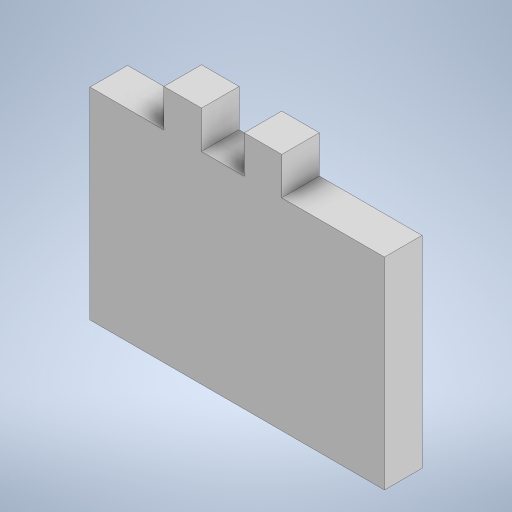
# Autodesk Inventor part: casterholderA
Saved by Autodesk Inventor 2023.2 (Build 272271000, 271)
## iProperties
Created: 2024-08-15
Part Number: casterholderA
Material: Generic
Document SubType Name: Modeling
Designer: PC
Density: 1 g/cm^3
Appearance: Default
Author: PC
Autodesk Inventor part; units mm, degrees
ref_plane "YZ Plane" through (0, 0, 0) normal (1, 0, 0) x (0, 1, 0)
ref_plane "XZ Plane" through (0, 0, 0) normal (0, 1, 0) x (-1, 0, 0)
ref_plane "XY Plane" through (0, 0, 0) normal (0, 0, 1) x (1, 0, 0)
sketch "Sketch1" plane through (0, 0, 0) normal (0, 0, 1) x (1, 0, 0)
  line L0 (20, -16.25) -> (-20, -16.25)
  line L1 (-20, -16.25) -> (-20, 16.25)
  line L2 (-20, 16.25) -> (20, 16.25)
  line L3 (20, 16.25) -> (20, -16.25)
  line L4 (20, -16.25) -> (-20, 16.25) construction
  line L5 (-20, -16.25) -> (20, 16.25) construction
  point P0 (0, 0)
  dimension "d0" = 40
  dimension "d1" = 32.5
  constraints: 12 end point, 2 midpoint, 2 parallel, 1 horizontal, 1 perpendicular
  measures "d0" distance of L1.end L2.end
  measures "d1" distance of L0.end L1.end
extrude "Extrusion1" add sketch "Sketch1" along normal blind 5.1
sketch "Sketch2" plane through (0, 0, 5.1) normal (0, 0, 1) x (1, 0, 0)
  line L0 (-20, 16.25) -> (-20, -16.25) projected
  line L1 (-20, 16.25) -> (-9.95, 16.25)
  line L2 (-9.95, 16.25) -> (-9.95, 11.15)
  line L3 (-9.95, 11.15) -> (-20, 11.15)
  line L4 (-20, 11.15) -> (-20, 16.25)
  line L5 (-4.85, 16.25) -> (0.95, 16.25)
  line L6 (0.95, 16.25) -> (0.95, 11.15)
  line L7 (0.95, 11.15) -> (-4.85, 11.15)
  line L8 (-4.85, 11.15) -> (-4.85, 16.25)
  line L9 (20, -16.25) -> (20, 16.25) projected
  line L10 (20, 16.25) -> (6.05, 16.25)
  line L11 (6.05, 16.25) -> (6.05, 11.15)
  line L12 (6.05, 11.15) -> (20, 11.15)
  line L13 (20, 11.15) -> (20, 16.25)
  line L14 (0, 0) -> (-4.3616, 0) construction
  dimension "d4" = 10.05
  dimension "d5" = 5.1
  dimension "d6" = 5.8
  dimension "d7" = 0.95
  dimension "d8" = 5.1
  dimension "d9" = 11.15
  dimension "d10" = 13.95
  constraints: 26 end point, 6 parallel, 4 horizontal, 3 perpendicular
  measures "d4" distance of L2.end L3.end
  measures "d5" distance of L1.end L2.end
  measures "d6" distance of L6.end L7.end
  measures "d7" distance from line of L14.start L6
  measures "d8" distance between parallel lines of L7 L5
  measures "d9" distance from line of L14.start L7
  measures "d10" distance of L12.end L11.end
extrude "Extrusion2" cut sketch "Sketch2" against normal blind 5.1
body "Solid1"
